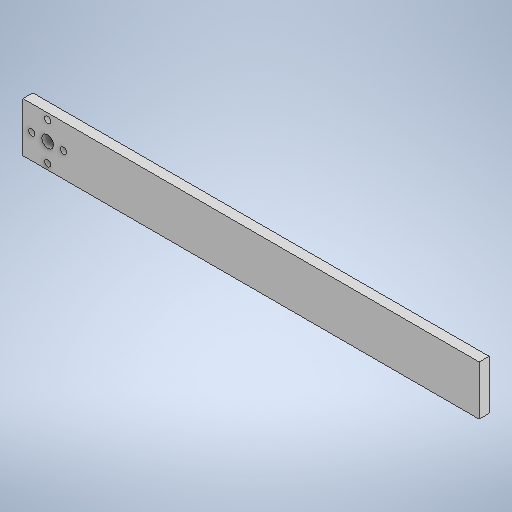
# Autodesk Inventor part: PeçaCerta
Saved by Autodesk Inventor 2025 (Build 290162000, 162)
## iProperties
Created: 2025-03-07
Part Number: PeçaCerta
Material: Genérico
Document SubType Name: Modeling
Designer: Ian
Density: 1 g/cm^3
Appearance: Padrão
Author: Ian
Autodesk Inventor part; units mm, degrees
ref_plane "YZ Plane" through (0, 0, 0) normal (1, 0, 0) x (0, 1, 0)
ref_plane "XZ Plane" through (0, 0, 0) normal (0, 1, 0) x (-1, 0, 0)
ref_plane "XY Plane" through (0, 0, 0) normal (0, 0, 1) x (1, 0, 0)
sketch "Esboço1" plane through (0, 0, 0) normal (0, 0, 1) x (1, 0, 0)
  circle A0 centre (12.5141, -8.1096) radius 1.6001
  circle A1 centre (20.5141, 1.3904) radius 1.6
  circle A2 centre (4.5141, 1.3904) radius 1.6
  circle A3 centre (12.5141, 1.3904) radius 3
  circle A4 centre (12.5141, 10.8904) radius 1.6
  line L0 (0.0141, 13.8904) -> (230.5141, 13.8904)
  line L1 (230.5141, 13.8904) -> (230.5141, -11.1096)
  line L2 (230.5141, -11.1096) -> (0.0141, -11.1096)
  line L3 (0.0141, -11.1096) -> (0.0141, 13.8904)
  line L4 (0.0141, 32.3338) -> (0.0141, -22.4463)
  point P0 (0, 0)
  point P1 (0.0141, 1.3904)
  dimension "d0" = 230.5
  dimension "d1" = 25
  dimension "d4" = 4.5
  dimension "d11" = 12.5
  dimension "d13" = 18.9999
  constraints: 10 end point, 5 centre point, 2 parallel, 2 vertical, 1 coincident, 1 collinear, 1 horizontal, 1 midpoint, 1 perpendicular
  measures "d0" distance of L1.end L2.end
  measures "d1" distance of L0.end L1.end
  measures "d4" distance of point (0.014, 1.39) A2.centre
  measures "d11" distance from line of L2 A2.centre
  measures "d13" distance of A4.centre A0.centre
extrude "Extrusão1" add sketch "Esboço1" along normal blind 5
